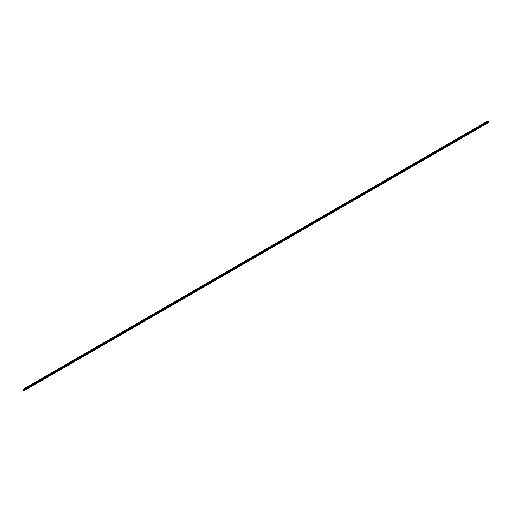
# Autodesk Inventor part: TL20240701-10100CV-GUIDE RAIL_H-21
Saved by Autodesk Inventor 2022.5 (Build 265521000, 521)
## iProperties
Category: PROFILE ASSY
Created: 2023-02-09
Part Number: TL20240701-10100CV-GUIDE RAIL_H-21
User Status: 1
Material: SS400
Description: 3
Document SubType Name: Modeling
Designer: 박성규
Density: 7.85 g/cm^3
Appearance: 일반 백색
DETAIL: Coveryor Assembly
M/C TITLE: CJ 제일제당 협동로봇 포장시스탬 PILOT 장비
PARTS NAME: Bracket
SPECIFICATION: TA20221101-CV200000-015
DocNumber: 221118_Standard_v1
Folder: .\
VDS_Category: 엔지니어링
Detail Description: Purchased products
Title: H-21-8540L
Author: 박성규
Revision Number: A
Autodesk Inventor part; units mm, degrees
ref_plane "YZ Plane" through (0, 0, 0) normal (1, 0, 0) x (0, 1, 0)
ref_plane "XZ Plane" through (0, 0, 0) normal (0, 1, 0) x (-1, 0, 0)
ref_plane "XY Plane" through (0, 0, 0) normal (0, 0, 1) x (1, 0, 0)
sketch "스케치9" plane through (0, 0, 0) normal (0, 0, 1) x (1, 0, 0)
  line L0 (-10.5, 5) -> (10.5, 5)
  line L1 (10.5, 5) -> (10.5, 0)
  line L2 (10.5, 0) -> (-10.5, 0)
  line L3 (-10.5, 0) -> (-10.5, 5)
  line L4 (-3.5, 0) -> (3.5, 0)
  line L5 (3.5, 0) -> (3.5, -4)
  line L6 (3.5, -4) -> (-3.5, -4)
  line L7 (-3.5, -4) -> (-3.5, 0)
  line L8 (-5.5, -4) -> (5.5, -4)
  line L9 (5.5, -4) -> (5.5, -6)
  line L10 (5.5, -6) -> (-5.5, -6)
  line L11 (-5.5, -6) -> (-5.5, -4)
  point P0 (0, 0)
  point P1 (0, 0)
  point P2 (0, -4)
  dimension "d40" = 11
  dimension "d41" = 21
  dimension "d42" = 7
  dimension "d43" = 5
  dimension "d44" = 4
  dimension "d45" = 2
  constraints: 24 end point, 6 parallel, 4 midpoint, 3 horizontal, 3 perpendicular, 1 coincident
  measures "d40" distance of L9.end L10.end
  measures "d41" distance of L0.start L0.end
  measures "d42" distance between parallel lines of L5 L7
  measures "d43" distance of L2.end L0.start
  measures "d44" distance between parallel lines of L8 L2
  measures "d45" distance of L10.end L8.start
extrude "돌출4" add sketch "스케치9" along normal mid plane 7680
equation "\"d46\" = L1 + L2"
equation "\"L1\" = 6000"
equation "\"L2\" = 1680"
